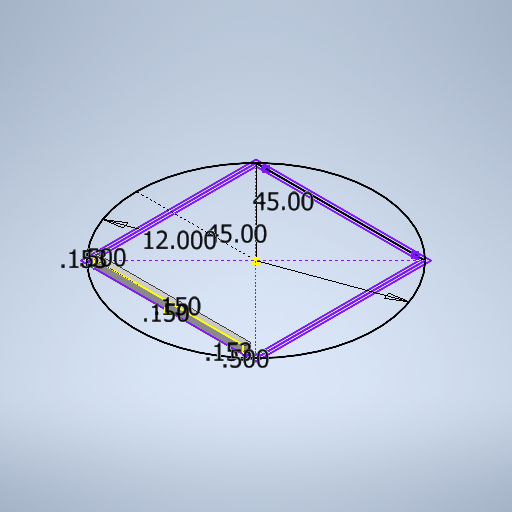
# Autodesk Inventor part: Base Disk Model
Saved by Autodesk Inventor 2025.1 (Build 291241000, 241)
## iProperties
Created: 2025-10-25
Part Number: Base Disk Model
Material: Generic
Document SubType Name: Modeling
Designer: benja
Density: 1 g/cm^3
Appearance: Anodized - Light Gray
Author: benja
Autodesk Inventor part; units mm, degrees
ref_plane "YZ Plane" through (0, 0, 0) normal (1, 0, 0) x (0, 1, 0)
ref_plane "XZ Plane" through (0, 0, 0) normal (0, 1, 0) x (-1, 0, 0)
ref_plane "XY Plane" through (0, 0, 0) normal (0, 0, 1) x (1, 0, 0)
sketch "Sketch3" plane through (0, 0, 0) normal (0, 1, 0) x (-1, 0, 0)
  circle A0 centre (0, 0) radius 152.4
  line L0 (0, 0) -> (107.7631, -107.7631)
  line L1 (0, 0) -> (152.4, 0) construction
  line L2 (107.7631, -107.7631) -> (-107.7631, -107.7631)
  line L3 (-107.7631, -107.7631) -> (-107.7631, 107.7631)
  line L4 (107.7631, 107.7631) -> (-107.7631, 107.7631)
  line L5 (-107.7631, 107.7631) -> (-107.7631, -107.7631)
  line L6 (-107.7631, -107.7631) -> (107.7631, -107.7631)
  line L7 (107.7631, -107.7631) -> (107.7631, 107.7631)
  line L8 (107.7631, 107.7631) -> (-107.7631, -107.7631) construction
  line L9 (-107.7631, 107.7631) -> (107.7631, -107.7631) construction
  line L10 (-111.5731, 111.5731) -> (111.5731, 111.5731)
  line L11 (111.5731, 111.5731) -> (111.5731, -111.5731)
  line L12 (111.5731, -111.5731) -> (-111.5731, -111.5731)
  line L13 (-111.5731, -111.5731) -> (-111.5731, 111.5731)
  line L14 (-103.9531, 103.9531) -> (103.9531, 103.9531)
  line L15 (103.9531, 103.9531) -> (103.9531, -103.9531)
  line L16 (103.9531, -103.9531) -> (-103.9531, -103.9531)
  line L17 (-103.9531, -103.9531) -> (-103.9531, 103.9531)
  line L18 (-107.7802, 107.7802) -> (107.7802, 107.7802)
  line L19 (107.7802, 107.7802) -> (107.7802, -107.7802)
  line L20 (107.7802, -107.7802) -> (-107.7802, -107.7802)
  line L21 (-107.7802, -107.7802) -> (-107.7802, 107.7802)
  line L22 (107.7802, 107.7802) -> (95.0802, 107.7802)
  line L23 (-107.7802, 107.7802) -> (-95.0802, 107.7802)
  line L24 (-95.0802, 107.7802) -> (95.0802, 107.7802) construction
  line L25 (-95.0802, 111.6074) -> (95.0802, 111.6074)
  line L26 (95.0802, 103.9531) -> (-95.0802, 103.9531)
  arc A1 (-95.0802, 111.6074) -> (-95.0802, 103.9531) centre (-95.0802, 107.7802) ccw
  arc A2 (95.0802, 103.9531) -> (95.0802, 111.6074) centre (95.0802, 107.7802) ccw
  arc A3 (-95.0802, -103.9531) -> (-95.0802, -111.6074) centre (-95.0802, -107.7802) ccw
  arc A4 (95.0802, -111.6074) -> (95.0802, -103.9531) centre (95.0802, -107.7802) ccw
  circle A5 centre (95.0802, 107.7802) radius 1.9431
  circle A6 centre (-95.0802, 107.7802) radius 1.9431
  point P0 (0, 107.7802)
  dimension "d31" = 304.8
  dimension "d32" = 45
  dimension "d33" = 45
  dimension "d34" = 3.81
  dimension "d35" = 3.81
  dimension "d36" = 12.7
  dimension "d37" = 12.7
  dimension "d38" = 3.8862
  dimension "d39" = 3.8862
  constraints: 56 end point, 11 point on circle, 9 parallel, 7 centre point, 6 symmetric about line, 4 perpendicular, 4 point on line, 4 tangent, 3 coincident, 3 midpoint, 2 horizontal, 1 collinear, 1 equal length, 11 other
  measures "d31" diameter of A0
  measures "d32" angle of L0 L1
  measures "d33" angle of L0 L2
  measures "d34" distance between parallel lines of L4 L10
  measures "d35" distance between parallel lines of L4 L14
  measures "d36" distance of L18.end L22.end
  measures "d37" distance of L18.start L23.end
  measures "d38" diameter of A5
  measures "d39" diameter of A6
extrude "Extrusion2" add sketch "Sketch3" along normal blind 10.16 contours A2 L14 A1 L4 A6 A5 | L4 A5 L18 A2 | A2 L18 A5 A6 A1 L10 | L10 A1 L25 A2 | A5 L4 | L4 A5 L18 | L18 A5 | L4 A6 L18 A5 | L18 A6 L4 A1 | A6 L4 | L4 A6 L18 | A6 L18
extrude "Extrusion3" cut sketch "Sketch3" along normal blind 10.16 contours A5 L4 | L4 A5 L18 | L18 A5 | A6 L4 | L4 A6 L18 | A6 L18
sketch "Sketch4" plane through (-95.0802, 0, 111.6074) normal (0, 0, 1) x (1, 0, 0)
  line L0 (0, 0) -> (190.1605, 0) projected
  line L1 (190.1605, 0) -> (190.1605, 10.16) projected
  line L2 (0, 10.16) -> (190.1605, 10.16) projected
  line L3 (0, 0) -> (0, 10.16) projected
  line L4 (0, 0) -> (0, 0) projected
  line L5 (0, 0) -> (0, 10.16) projected
  line L6 (0, 10.16) -> (0, 10.16) projected
  line L7 (0, 0) -> (0, 10.16) projected
  line L8 (190.1605, 0) -> (190.1605, 0) projected
  line L9 (190.1605, 0) -> (190.1605, 10.16) projected
  line L10 (190.1605, 10.16) -> (190.1605, 10.16) projected
  line L11 (190.1605, 0) -> (190.1605, 10.16) projected
  line L12 (0, 10.16) -> (-3.8272, 10.16) projected
  line L13 (0, 5.08) -> (-3.8272, 5.08)
  line L14 (-3.8272, 5.08) -> (-3.8272, 10.16)
  line L15 (-3.8272, 10.16) -> (0, 10.16)
  line L16 (0, 10.16) -> (0, 5.08)
  point P0 (95.0802, 0)
  constraints: 8 end point, 2 parallel, 1 horizontal, 1 midpoint, 1 perpendicular
body "Solid2"
